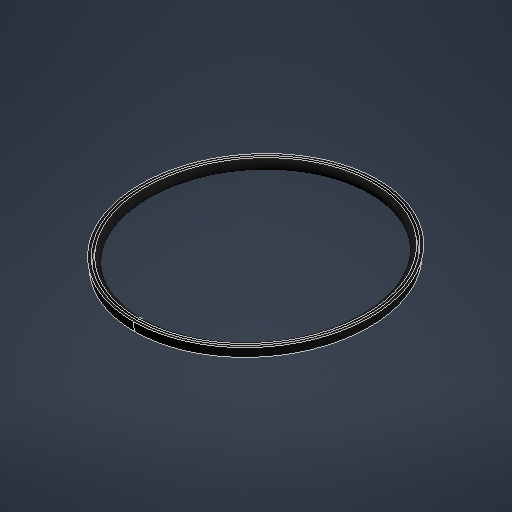
# Autodesk Inventor part: BOTTOM_ELIP_BEARING_SEAL,REV-ENG
Saved by Autodesk Inventor 2026.2 (Build 302298010, 298A)
## iProperties
Created: 2026-03-06
Part Number: BOTTOM_ELIP_BEARING_SEAL,REV-ENG
Material: Polyethylene, UHMW
Document SubType Name: Modeling
Designer: 4aida
Density: 0.930045 g/cm^3
Appearance: Black
Author: 4aida
Autodesk Inventor part; units mm, degrees
ref_plane "YZ Plane" through (0, 0, 0) normal (1, 0, 0) x (0, 1, 0)
ref_plane "XZ Plane" through (0, 0, 0) normal (0, 1, 0) x (-1, 0, 0)
ref_plane "XY Plane" through (0, 0, 0) normal (0, 0, 1) x (1, 0, 0)
sketch "Sketch1" plane through (0, 0, 0) normal (0, 1, 0) x (-1, 0, 0)
  ellipse E0 centre (0, 0) end of major axis (0, 15.7) minor radius 14.7
  dimension "d0" = 15.7
  dimension "d1" = 14.7
  constraints: 1 coincident, 2 other
sketch "Sketch2" plane through (0, 0, 0) normal (1, 0, 0) x (0, 1, 0)
  line L0 (0, -15.7) -> (0, 15.7) construction
  line L1 (-0.625, -15.7) -> (-0.625, -16.2104)
  line L2 (-0.625, -16.2104) -> (0.625, -16.375)
  line L3 (0.625, -16.375) -> (0.625, -16.022)
  line L4 (0.625, -16.022) -> (-0.325, -15.8969)
  line L5 (-0.325, -15.8969) -> (0.625, -15.7)
  arc A0 (0.625, -15.7) -> (-0.625, -15.7) centre (0, -15.7) ccw
  point P0 (0, 0)
  point P1 (0, -15.075)
  dimension "d5" = 0.625
  dimension "d6" = 1.3
  dimension "d7" = 0.35
  dimension "d8" = 97.5
  dimension "d9" = 0.3
  constraints: 10 end point, 3 point on circle, 3 vertical alignment, 2 vertical, 1 centre point, 1 coincident, 1 parallel, 1 tangent
  measures "d5" radius of A0
  measures "d6" vertical distance of L2.end point (0, -15.075)
  measures "d7" distance between parallel lines of L2 L4
  measures "d8" angle of L2 L1
  measures "d9" distance from line of L1 L4.end
sweep "Sweep1" add profiles "Sketch2" path "Sketch1"
body "Solid1"
